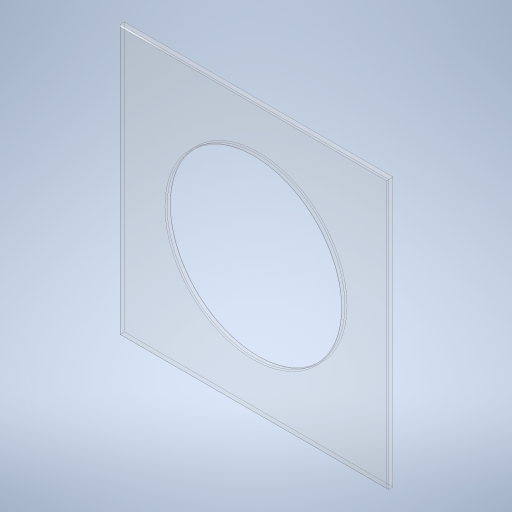
# Autodesk Inventor part: groundPlateWoodV1
Saved by Autodesk Inventor 2024.4 (Build 284460000, 460)
## iProperties
Created: 2025-11-05
Part Number: groundPlateWoodV1
Material: PMMA Plastic
Document SubType Name: Modeling
Designer: jonas
Density: 1.188 g/cm^3
Appearance: Polycarbonate - Clear
Author: jonas
Autodesk Inventor part; units mm, degrees
ref_plane "YZ Plane" through (0, 0, 0) normal (1, 0, 0) x (0, 1, 0)
ref_plane "XZ Plane" through (0, 0, 0) normal (0, 1, 0) x (-1, 0, 0)
ref_plane "XY Plane" through (0, 0, 0) normal (0, 0, 1) x (1, 0, 0)
sketch "Sketch1" plane through (0, 0, 0) normal (0, 1, 0) x (-1, 0, 0)
  line L0 (0, -102.1042) -> (0, 102.1042) construction
  line L1 (37.5532, 0) -> (-37.5532, 0) construction
  line L2 (500, 500) -> (-500, 500)
  line L3 (-500, 500) -> (-500, -500)
  line L4 (-500, -500) -> (500, -500)
  line L5 (500, -500) -> (500, 500)
  circle A0 centre (0, 0) radius 325
  dimension "d0" = 1000
  dimension "d1" = 1000
  dimension "d2" = 650
  constraints: 12 end point, 2 coincident, 2 horizontal, 2 midpoint, 2 parallel, 1 centre point, 1 perpendicular, 1 vertical, 2 other
  measures "d0" distance between parallel lines of L2 L4
  measures "d1" distance between parallel lines of L3 L5
  measures "d2" diameter of A0
extrude "Extrusion1" add sketch "Sketch1" along normal blind 20
chamfer "Chamfer1" distance 4 angle 45 6 edges at (325, 20, 0) (325, 0, 0) (-500, 0, 0) (0, 0, 500) (0, 0, -500) (500, 0, 0)
body "Solid1"
